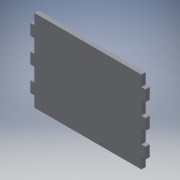
# Autodesk Inventor part: Bottom
Saved by Autodesk Inventor 2018 (Build 220112000, 112)
## iProperties
Created: 2017-10-30
Part Number: Bottom
Material: Polycarbonate, Clear
Document SubType Name: Modeling
Designer: xl0
Density: 1.2 g/cm^3
Appearance: Polycarbonate - Clear
Author: xl0
Autodesk Inventor part; units mm, degrees
ref_plane "YZ Plane" through (0, 0, 0) normal (1, 0, 0) x (0, 1, 0)
ref_plane "XZ Plane" through (0, 0, 0) normal (0, 1, 0) x (-1, 0, 0)
ref_plane "XY Plane" through (0, 0, 0) normal (0, 0, 1) x (1, 0, 0)
sketch "Sketch1" plane through (0, 0, 0) normal (0, 0, 1) x (1, 0, 0)
  line L0 (-79, -26.3395) -> (-79, 33.1605) projected
  line L1 (-1.5, -26.3395) -> (-79, -26.3395) projected
  line L2 (-1.5, -9.5895) -> (-1.5, -26.3395) projected
  line L3 (-1.5, 8.4105) -> (-1.5, -1.5895) projected
  line L4 (-1.5, 33.1605) -> (-1.5, 16.4105) projected
  line L5 (-79, 33.1605) -> (-1.5, 33.1605) projected
  line L6 (-1.5, -9.5895) -> (-1.5, -1.5895)
  line L7 (-1.5, 8.4105) -> (-1.5, 16.7071)
  line L8 (-74, -21.3395) -> (-60.5, -21.3395) construction
  line L9 (-74, -7.8395) -> (-74, -21.3395) construction
  line L10 (-60.5, -7.8395) -> (-74, -7.8395) construction
  line L11 (-60.5, -21.3395) -> (-60.5, -7.8395) construction
  line L12 (-74, -3.3395) -> (-60.5, -3.3395) construction
  line L13 (-74, 10.1605) -> (-74, -3.3395) construction
  line L14 (-60.5, 10.1605) -> (-74, 10.1605) construction
  line L15 (-60.5, 10.1605) -> (-74, 10.1605) construction
  line L16 (-60.5, -3.3395) -> (-60.5, 10.1605) construction
  line L17 (-74, 14.6605) -> (-60.5, 14.6605) construction
  line L18 (-74, 28.1605) -> (-74, 14.6605) construction
  line L19 (-60.5, 28.1605) -> (-74, 28.1605) construction
  line L20 (-60.5, 14.6605) -> (-60.5, 28.1605) construction
  line L21 (-79, -18.5895) -> (-82, -18.5895)
  line L22 (-82, -18.5895) -> (-82, -10.5895)
  line L23 (-82, -10.5895) -> (-79, -10.5895)
  line L24 (-79, -0.5895) -> (-82, -0.5895)
  line L25 (-82, -0.5895) -> (-82, 7.4105)
  line L26 (-82, 7.4105) -> (-79, 7.4105)
  line L27 (-79, 17.4105) -> (-82, 17.4105)
  line L28 (-82, 17.4105) -> (-82, 25.4105)
  line L29 (-82, 25.4105) -> (-79, 25.4105)
  line L30 (-82, -9.5895) -> (-82, -1.5895) construction
  line L31 (1.5, -1.5895) -> (1.5, -9.5895) construction
  line L32 (-10.3701, -14.5895) -> (-89.08, -14.5895) construction
  line L33 (-89.5983, 3.4105) -> (-12.2572, 3.4105) construction
  line L34 (-89.5983, 21.4105) -> (-12.2572, 21.4105) construction
  line L35 (-1.5, -18.5895) -> (1.5, -18.5895)
  line L36 (1.5, -18.5895) -> (1.5, -10.5895)
  line L37 (1.5, -10.5895) -> (-1.5, -10.5895)
  line L38 (-1.5, -0.5895) -> (1.5, -0.5895)
  line L39 (1.5, -0.5895) -> (1.5, 7.4105)
  line L40 (1.5, 7.4105) -> (-1.5, 7.4105)
  line L41 (-1.5, 17.4105) -> (1.5, 17.4105)
  line L42 (1.5, 17.4105) -> (1.5, 25.4105)
  line L43 (1.5, 25.4105) -> (-1.5, 25.4105)
  point P0 (0, 0)
  point P1 (-74, -14.5895)
  point P2 (-74, 3.4105)
  point P3 (-74, 21.4105)
  point P4 (-82, -14.5895)
  point P5 (-82, 3.4105)
  point P6 (-82, 21.4105)
  point P7 (1.5, -14.5895)
  point P8 (1.5, 3.4105)
  point P9 (1.5, 21.4105)
  constraints: 46 end point, 24 point on line, 11 perpendicular, 9 midpoint, 6 equal length, 5 vertical, 4 collinear, 4 horizontal, 2 parallel
extrude "Extrusion1" add sketch "Sketch1" against normal blind 3
body "Solid1"
